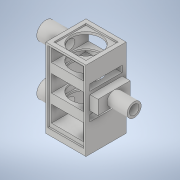
# Autodesk Inventor part: HDAcell_Daniela_thickelecrode_08172020
Saved by Autodesk Inventor 2020.3 (Build 243373000, 373)
## iProperties
Created: 2020-02-08
Part Number: HDAcell_Daniela_thickelecrode_08172020
Material: Generic
Document SubType Name: Modeling
Designer: Quinten
Density: 1 g/cm^3
Appearance: Default
Author: Quinten
Autodesk Inventor part; units mm, degrees
ref_plane "YZ Plane" through (0, 0, 0) normal (1, 0, 0) x (0, 1, 0)
ref_plane "XZ Plane" through (0, 0, 0) normal (0, 1, 0) x (-1, 0, 0)
ref_plane "XY Plane" through (0, 0, 0) normal (0, 0, 1) x (1, 0, 0)
sketch "Sketch1" plane through (0, 0, 0) normal (0, 1, 0) x (-1, 0, 0)
  line L0 (0, 0) -> (20, 0)
  line L1 (20, 0) -> (20, 20)
  line L2 (20, 20) -> (0, 20)
  line L3 (0, 20) -> (0, 0)
  dimension "d0" = 20
  dimension "d1" = 20
  constraints: 8 end point, 2 parallel, 1 horizontal, 1 perpendicular
  measures "d0" distance between parallel lines of L3 L1
  measures "d1" distance between parallel lines of L0 L2
extrude "Extrusion1" add sketch "Sketch1" along normal blind 34.4
sketch "Sketch2" plane through (0, 34.4, 0) normal (0, 1, 0) x (1, 0, 0)
  circle A0 centre (-10, -10) radius 7.5
  line L0 (0, 0) -> (-20, 0) projected
  line L1 (0, -20) -> (0, 0) projected
  dimension "d4" = 10
  dimension "d5" = 10
  dimension "d6" = 15
  constraints: 1 centre point
  measures "d4" distance from line of L0 A0.centre
  measures "d5" distance from line of L1 A0.centre
  measures "d6" diameter of A0
extrude "Extrusion2" cut sketch "Sketch2" against normal blind 30
sketch "Sketch3" plane through (0, 0, 20) normal (1, 0, 0) x (0, 0, -1)
  line L0 (2, 12.2) -> (18, 12.2)
  line L1 (18, 12.2) -> (18, 9)
  line L2 (18, 9) -> (2, 9)
  line L3 (2, 9) -> (2, 12.2)
  line L4 (20, 0) -> (20, 34.4) projected
  line L5 (0, 0) -> (20, 0) projected
  dimension "d9" = 3.2
  dimension "d12" = 16
  dimension "d13" = 2
  dimension "d14" = 9
  constraints: 8 end point, 2 parallel, 1 horizontal, 1 perpendicular
  measures "d9" distance between parallel lines of L0 L2
  measures "d12" distance between parallel lines of L1 L3
  measures "d13" distance between parallel lines of L4 L1
  measures "d14" distance between parallel lines of L5 L2
extrude "Extrusion3" cut sketch "Sketch3" against normal blind 18
sketch "Sketch4" plane through (0, 0, 20) normal (1, 0, 0) x (0, 0, -1)
  line L0 (2, 25.4) -> (18, 25.4)
  line L1 (18, 25.4) -> (18, 22.2)
  line L2 (18, 22.2) -> (2, 22.2)
  line L3 (2, 22.2) -> (2, 25.4)
  line L4 (20, 0) -> (20, 34.4) projected
  line L5 (0, 0) -> (20, 0) projected
  line L6 (2, 12.2) -> (18, 12.2) projected
  dimension "d17" = 2
  dimension "d18" = 16
  dimension "d19" = 3.2
  dimension "d21" = 10
  constraints: 8 end point, 2 parallel, 1 horizontal, 1 perpendicular
  measures "d17" distance between parallel lines of L4 L1
  measures "d18" distance between parallel lines of L3 L1
  measures "d19" distance between parallel lines of L0 L2
  measures "d21" distance between parallel lines of L6 L2
extrude "Extrusion4" cut sketch "Sketch4" against normal blind 18
sketch "Sketch5" plane through (0, 34.4, 0) normal (0, 1, 0) x (1, 0, 0)
  line L0 (-18, -18) -> (-2, -18)
  line L1 (-2, -18) -> (-2, -2)
  line L2 (-2, -2) -> (-18, -2)
  line L3 (-18, -2) -> (-18, -18)
  line L4 (-20, 0) -> (-20, -20) projected
  line L5 (-20, -20) -> (0, -20) projected
  line L6 (0, -20) -> (0, 0) projected
  line L7 (0, 0) -> (-20, 0) projected
  dimension "d24" = 2
  dimension "d25" = 2
  dimension "d26" = 2
  dimension "d27" = 2
  constraints: 8 end point, 2 parallel, 1 horizontal, 1 perpendicular
  measures "d24" distance between parallel lines of L4 L3
  measures "d25" distance between parallel lines of L5 L0
  measures "d26" distance between parallel lines of L6 L1
  measures "d27" distance between parallel lines of L7 L2
extrude "Extrusion5" cut sketch "Sketch5" against normal blind 0.8 contours L3 L2 L1 L0
sketch "Sketch10" plane through (0, 0, 20) normal (1, 0, 0) x (0, 0, -1)
  line L0 (2, 20.2) -> (18, 20.2)
  line L1 (18, 20.2) -> (18, 14.2)
  line L2 (18, 14.2) -> (2, 14.2)
  line L3 (2, 14.2) -> (2, 20.2)
  line L4 (18, 22.2) -> (2, 22.2) projected
  line L5 (0, 0) -> (0, 34.4) projected
  line L6 (2, 12.2) -> (18, 12.2) projected
  line L7 (20, 0) -> (20, 34.4) projected
  dimension "d46" = 2
  dimension "d47" = 2
  dimension "d48" = 2
  dimension "d49" = 2
  constraints: 8 end point, 2 parallel, 1 horizontal, 1 perpendicular
  measures "d46" distance between parallel lines of L4 L0
  measures "d47" distance between parallel lines of L5 L3
  measures "d48" distance between parallel lines of L6 L2
  measures "d49" distance between parallel lines of L7 L1
extrude "Extrusion7" cut sketch "Sketch10" against normal blind 17.5
sketch "Sketch6" plane through (0, 0, 20) normal (1, 0, 0) x (0, 0, -1)
  line L0 (2, 20.7) -> (18, 20.7)
  line L1 (18, 20.7) -> (18, 13.7)
  line L2 (18, 13.7) -> (2, 13.7)
  line L3 (2, 13.7) -> (2, 20.7)
  line L4 (0, 0) -> (0, 34.4) projected
  line L5 (20, 0) -> (20, 34.4) projected
  line L6 (18, 22.2) -> (2, 22.2) projected
  line L7 (2, 12.2) -> (18, 12.2) projected
  dimension "d30" = 2
  dimension "d31" = 2
  dimension "d32" = 1.5
  dimension "d33" = 1.5
  constraints: 8 end point, 2 parallel, 1 horizontal, 1 perpendicular
  measures "d30" distance between parallel lines of L4 L3
  measures "d31" distance between parallel lines of L5 L1
  measures "d32" distance between parallel lines of L6 L0
  measures "d33" distance between parallel lines of L7 L2
extrude "Extrusion6" add sketch "Sketch6" along normal blind 4
sketch "Sketch7" plane through (4, 0, 20) normal (1, 0, 0) x (0, 0, -1)
  circle A0 centre (10, 17.2) radius 2.4
  line L0 (18, 20.7) -> (2, 20.7) projected
  line L1 (18, 13.7) -> (18, 20.7) projected
  point P0 (20, 0)
  dimension "d36" = 4.8
  dimension "d37" = 3.5
  dimension "d38" = 8
  constraints: 1 centre point
  measures "d36" diameter of A0
  measures "d37" distance from line of L0 A0.centre
  measures "d38" distance from line of L1 A0.centre
loft "Loft2" cut profiles "Sketch10", "Sketch7"
sketch "Sketch11" plane through (4, 0, 20) normal (1, 0, 0) x (0, 0, -1)
  circle A0 centre (10, 17.2) radius 3.5
  line L0 (2, 13.7) -> (18, 13.7) projected
  line L1 (18, 13.7) -> (18, 20.7) projected
  point P0 (20, 0)
  dimension "d56" = 7
  dimension "d57" = 3.5
  dimension "d58" = 8
  constraints: 1 centre point
  measures "d56" diameter of A0
  measures "d57" distance from line of L0 A0.centre
  measures "d58" distance from line of L1 A0.centre
extrude "Extrusion8" add sketch "Sketch11" along normal blind 10
sketch "Sketch12" plane through (14, 17.2, 10) normal (1, 0, 0) x (0, 0, -1)
  circle A0 centre (0, 0) radius 2.4
  circle A1 centre (0, 0) radius 3.5 projected
  line L0 (8, -3.5) -> (8, 3.5) projected
  point P0 (10, -17.2)
  dimension "d62" = 4.8
  dimension "d63" = 0
  dimension "d64" = 8
  constraints: 1 centre point
  measures "d62" diameter of A0
  measures "d63" distance of A1.centre A0.centre
  measures "d64" distance from line of L0 A0.centre
extrude "Extrusion9" cut sketch "Sketch12" against normal blind 10 contours A0
sketch "Sketch13" plane through (-20, 0, 0) normal (-1, 0, 0) x (0, 0, 1)
  circle A0 centre (10, 4.4) radius 4.5
  line L0 (0, 0) -> (0, 34.4) projected
  line L1 (0, 0) -> (20, 0) projected
  dimension "d67" = 9
  dimension "d68" = 10
  dimension "d69" = 4.4
  constraints: 1 centre point
  measures "d67" diameter of A0
  measures "d68" distance from line of L0 A0.centre
  measures "d69" distance from line of L1 A0.centre
sketch "Sketch14" plane through (-20, 0, 0) normal (-1, 0, 0) x (0, 0, 1)
  circle A0 centre (10, 4.4) radius 2.4
  line L0 (20, 0) -> (20, 34.4) projected
  line L1 (0, 0) -> (0, 34.4) projected
  line L2 (0, 0) -> (20, 0) projected
  dimension "d71" = 10
  dimension "d72" = 4.4
  dimension "d90" = 4.8
  constraints: 1 centre point
  measures "d71" distance from line of L1 A0.centre
  measures "d72" distance from line of L2 A0.centre
  measures "d90" diameter of A0
extrude "Extrusion10" cut sketch "Sketch14" against normal blind 4
extrude "Extrusion11" add sketch "Sketch13" along normal blind 10
sketch "Sketch15" plane through (-30, 4.4, 10) normal (-1, 0, 0) x (0, 0, 1)
  circle A0 centre (0, 0) radius 2.4
  point P0 (-10, -4.4)
  dimension "d77" = 4.8
  constraints: 1 centre point
  measures "d77" diameter of A0
extrude "Extrusion12" cut sketch "Sketch15" against normal blind 10
sketch "Sketch16" plane through (-20, 0, 20) normal (-1, 0, 0) x (0, 0, 1)
  circle A0 centre (-10, 29.4) radius 4.5
  line L0 (0, 0) -> (0, 34.4) projected
  line L1 (-20, 34.4) -> (0, 34.4) projected
  point P0 (-20, 0)
  dimension "d80" = 10
  dimension "d81" = 5
  dimension "d82" = 9
  constraints: 1 centre point
  measures "d80" distance from line of L0 A0.centre
  measures "d81" distance from line of L1 A0.centre
  measures "d82" diameter of A0
extrude "Extrusion13" add sketch "Sketch16" along normal blind 10
sketch "Sketch17" plane through (-30, 29.4, 10) normal (-1, 0, 0) x (0, 0, 1)
  circle A0 centre (0, 0) radius 2.4
  point P0 (-10, -29.4)
  dimension "d85" = 4.8
  constraints: 1 centre point
  measures "d85" diameter of A0
extrude "Extrusion14" cut sketch "Sketch17" against normal blind 14
sketch "Sketch18" plane through (0, 0, 0) normal (0, -1, 0) x (1, 0, 0)
  line L0 (-20, 20) -> (0, 20) projected
  line L1 (0, 20) -> (0, 0) projected
  line L2 (-20, 20) -> (0, 20)
  line L3 (0, 20) -> (0, 0)
  line L4 (0, 0) -> (-20, 0)
  line L5 (-20, 0) -> (-20, 20)
  constraints: 8 end point, 2 parallel, 1 horizontal, 1 perpendicular
extrude "Extrusion15" add sketch "Sketch18" along normal blind 5
sketch "Sketch19" plane through (-20, 34.4, 20) normal (0, 0, 1) x (1, 0, 0)
  line L0 (2, -26.2) -> (18, -26.2)
  line L1 (18, -26.2) -> (18, -34.4)
  line L2 (18, -34.4) -> (2, -34.4)
  line L3 (2, -34.4) -> (2, -26.2)
  line L4 (20, -39.4) -> (0, -39.4) projected
  line L5 (20, -39.4) -> (20, 0) projected
  line L6 (0, -39.4) -> (0, 0) projected
  point P0 (20, -34.4)
  dimension "d91" = 13.2
  dimension "d92" = 5
  dimension "d93" = 2
  dimension "d94" = 2
  constraints: 8 end point, 2 parallel, 1 horizontal, 1 perpendicular
  measures "d91" distance between parallel lines of L4 L0
  measures "d92" distance between parallel lines of L4 L2
  measures "d93" distance between parallel lines of L5 L1
  measures "d94" distance between parallel lines of L6 L3
extrude "Extrusion16" cut sketch "Sketch19" against normal blind 20
sketch "Sketch20" plane through (-20, 34.4, 20) normal (0, 0, 1) x (1, 0, 0)
  line L0 (18, -21.4) -> (2, -21.4)
  line L1 (2, -21.4) -> (2, -13)
  line L2 (2, -13) -> (18, -13)
  line L3 (18, -13) -> (18, -21.4)
  line L4 (0, -39.4) -> (0, 0) projected
  line L5 (20, -39.4) -> (20, 0) projected
  line L6 (20, -39.4) -> (0, -39.4) projected
  point P0 (20, -34.4)
  dimension "d97" = 2
  dimension "d98" = 2
  dimension "d99" = 18
  dimension "d100" = 8.4
  constraints: 8 end point, 2 parallel, 1 horizontal, 1 perpendicular
  measures "d97" distance between parallel lines of L4 L1
  measures "d98" distance between parallel lines of L5 L3
  measures "d99" distance between parallel lines of L6 L0
  measures "d100" distance between parallel lines of L0 L2
extrude "Extrusion17" cut sketch "Sketch20" against normal blind 20
sketch "Sketch21" plane through (-20, 34.4, 20) normal (0, 0, 1) x (1, 0, 0)
  line L0 (18, -8.2) -> (2, -8.2)
  line L1 (2, -8.2) -> (2, -2)
  line L2 (2, -2) -> (18, -2)
  line L3 (18, -2) -> (18, -8.2)
  line L4 (20, -39.4) -> (20, 0) projected
  line L5 (0, -39.4) -> (0, 0) projected
  line L6 (0, 0) -> (20, 0) projected
  point P0 (20, -34.4)
  dimension "d103" = 2
  dimension "d104" = 2
  dimension "d105" = 2
  dimension "d106" = 8.2
  constraints: 8 end point, 2 parallel, 1 horizontal, 1 perpendicular
  measures "d103" distance between parallel lines of L4 L3
  measures "d104" distance between parallel lines of L5 L1
  measures "d105" distance between parallel lines of L6 L2
  measures "d106" distance between parallel lines of L6 L0
extrude "Extrusion18" cut sketch "Sketch21" against normal blind 20
sketch "Sketch22" plane through (-20, 34.4, 20) normal (0, 0, 1) x (1, 0, 0)
  line L0 (1, -1) -> (19, -1)
  line L1 (19, -1) -> (19, -36.4)
  line L2 (19, -36.4) -> (1, -36.4)
  line L3 (1, -36.4) -> (1, -1)
  line L4 (0, 0) -> (20, 0) projected
  line L5 (20, -39.4) -> (20, 0) projected
  line L6 (0, -39.4) -> (0, 0) projected
  line L7 (18, -34.4) -> (2, -34.4) projected
  point P0 (20, -34.4)
  dimension "d109" = 1
  dimension "d110" = 1
  dimension "d112" = 1
  dimension "d115" = 2
  constraints: 8 end point, 2 parallel, 1 horizontal, 1 perpendicular
  measures "d109" distance between parallel lines of L4 L0
  measures "d110" distance between parallel lines of L5 L1
  measures "d112" distance between parallel lines of L6 L3
  measures "d115" distance between parallel lines of L7 L2
extrude "Extrusion19" cut sketch "Sketch22" against normal blind 0.8
sketch "Sketch23" plane through (0, 34.4, 0) normal (0, 0, -1) x (-1, 0, 0)
  line L0 (1, -36.4) -> (19, -36.4)
  line L1 (19, -36.4) -> (19, -1)
  line L2 (19, -1) -> (1, -1)
  line L3 (1, -1) -> (1, -36.4)
  line L4 (0, 0) -> (20, 0) projected
  line L5 (0, 0) -> (0, -39.4) projected
  line L6 (20, -39.4) -> (20, 0) projected
  line L7 (18, -34.4) -> (2, -34.4) projected
  point P0 (0, -34.4)
  dimension "d116" = 1
  dimension "d117" = 1
  dimension "d118" = 1
  dimension "d119" = 2
  constraints: 8 end point, 2 parallel, 1 horizontal, 1 perpendicular
  measures "d116" distance between parallel lines of L4 L2
  measures "d117" distance between parallel lines of L5 L3
  measures "d118" distance between parallel lines of L6 L1
  measures "d119" distance between parallel lines of L7 L0
extrude "Extrusion20" cut sketch "Sketch23" against normal blind 0.8
body "Solid1"
